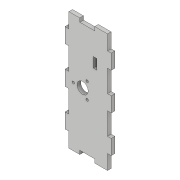
# Autodesk Inventor part: costat3
Saved by Autodesk Inventor 2019 (Build 230136000, 136)
## iProperties
Created: 2018-09-21
Part Number: costat3
Material: Genérico
Document SubType Name: Modeling
Designer: lmacia
Density: 1 g/cm^3
Appearance: Valor por defecto
Author: lmacia
Autodesk Inventor part; units mm, degrees
ref_plane "YZ Plane" through (0, 0, 0) normal (1, 0, 0) x (0, 1, 0)
ref_plane "XZ Plane" through (0, 0, 0) normal (0, 1, 0) x (-1, 0, 0)
ref_plane "XY Plane" through (0, 0, 0) normal (0, 0, 1) x (1, 0, 0)
sketch "Boceto1" plane through (0, 0, 0) normal (0, 0, 1) x (-1, 0, 0)
  line L0 (-18.5763, -36.3749) -> (-15.5263, -36.3749)
  line L1 (-15.5263, -36.3749) -> (-15.5263, -48.4733)
  line L2 (-15.5263, -48.4733) -> (-5.0037, -48.4733)
  line L3 (-5.0037, -48.4733) -> (-5.0037, -45.4233)
  line L4 (-5.0037, -45.4233) -> (7.1965, -45.4233)
  line L5 (7.1965, -45.4233) -> (7.1965, -48.4733)
  line L6 (7.1965, -48.4733) -> (9.5287, -48.4733)
  line L7 (9.5287, -48.4733) -> (16.194, -48.4733)
  line L8 (16.194, -48.4733) -> (16.194, -47.9303)
  line L9 (16.194, -47.9303) -> (16.194, -45.4233)
  line L10 (16.194, -45.4233) -> (16.194, -36.3411)
  line L11 (16.194, -36.3411) -> (19.2441, -36.3411)
  line L12 (19.2441, -36.3411) -> (19.2441, -24.1748)
  line L13 (19.2444, -24.1748) -> (16.1963, -24.1748)
  line L14 (16.1963, -24.1748) -> (16.1954, -10.116)
  line L15 (16.1954, -10.116) -> (16.194, -6.0779)
  line L16 (16.1918, -6.1454) -> (16.194, -6.0779)
  line L17 (16.194, -6.0779) -> (19.2441, -6.0779)
  line L18 (19.2441, -6.0779) -> (19.2441, 6.1222)
  line L19 (19.2441, 6.1222) -> (16.194, 6.1222)
  line L20 (16.194, 6.1222) -> (16.194, 24.2191)
  line L21 (16.194, 24.2191) -> (19.2441, 24.2191)
  line L22 (19.2441, 24.2191) -> (19.2441, 36.4192)
  line L23 (19.2441, 36.4192) -> (16.194, 36.4192)
  line L24 (16.194, 36.4192) -> (16.194, 45.4676)
  line L25 (16.194, 45.4676) -> (16.194, 48.5176)
  line L26 (16.194, 48.5176) -> (7.1965, 48.5176)
  line L27 (7.1965, 48.5176) -> (7.1965, 45.4676)
  line L28 (7.1965, 45.4676) -> (-3.3262, 45.4676)
  line L29 (-3.3262, 45.4676) -> (-5.0037, 45.4676)
  line L30 (-5.0037, 45.4676) -> (-5.0037, 48.5176)
  line L31 (-5.0037, 48.5176) -> (-15.5263, 48.5176)
  line L32 (-15.5263, 48.5176) -> (-15.5263, 36.4192)
  line L33 (-15.5263, 36.4192) -> (-18.5763, 36.4192)
  line L34 (-18.5763, 36.4192) -> (-18.5763, 24.2191)
  line L35 (-18.5763, 24.2191) -> (-15.5263, 24.2191)
  line L36 (-15.5263, 24.2191) -> (-15.5263, 6.1222)
  line L37 (-15.5263, 6.1222) -> (-18.5763, 6.1222)
  line L38 (-18.5763, 6.1222) -> (-18.5763, -6.0779)
  line L39 (-18.5763, -6.0779) -> (-15.5263, -6.0779)
  line L40 (-15.5263, -6.0779) -> (-15.5263, -24.1748)
  line L41 (-15.5263, -24.1748) -> (-17.5596, -24.1748)
  line L42 (-17.5596, -24.1748) -> (-18.5763, -24.1748)
  line L43 (-18.5763, -24.1748) -> (-18.5763, -36.3749)
  line L44 (-16.0528, -24.1739) -> (-19.1028, -24.1739)
  line L45 (6.6699, 45.4684) -> (4.9416, 45.4684)
  line L46 (-3.8527, -18.4805) -> (-3.8527, -26.614)
  line L47 (-3.8527, -26.614) -> (-6.9027, -26.614)
  line L48 (-6.9027, -26.614) -> (-6.9027, -18.4805)
  line L49 (-6.9027, -18.4805) -> (-3.8527, -18.4805)
  circle A0 centre (1.129, 6.6314) radius 1.0167
  circle A1 centre (4.8907, 0.023) radius 4.575
  circle A2 centre (12.5158, 0.023) radius 1.0167
  circle A3 centre (1.129, -6.5854) radius 1.0167
  point P0 (0, 0)
  dimension "d2" = 96.991
  dimension "d3" = 37.82
  constraints: 100 end point, 4 centre point, 1 horizontal, 1 point on line
  measures "d2" distance between parallel lines of L26 L7
extrude "Extrusión1" add sketch "Boceto1" along normal blind 3
